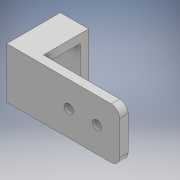
# Autodesk Inventor part: Wheel Holder Rev 2
Saved by Autodesk Inventor 2018 (Build 220112000, 112)
## iProperties
Created: 2018-05-04
Part Number: Wheel Holder Rev 2
Material: Generic
Document SubType Name: Modeling
Designer: alexs
Density: 1 g/cm^3
Appearance: Default
Author: alexs
Autodesk Inventor part; units mm, degrees
ref_plane "YZ Plane" through (0, 0, 0) normal (1, 0, 0) x (0, 1, 0)
ref_plane "XZ Plane" through (0, 0, 0) normal (0, 1, 0) x (-1, 0, 0)
ref_plane "XY Plane" through (0, 0, 0) normal (0, 0, 1) x (1, 0, 0)
sketch "Sketch1" plane through (0, 0, 0) normal (1, 0, 0) x (0, 1, 0)
  line L0 (0, 0) -> (10, 0)
  line L1 (10, 0) -> (10, -12)
  line L2 (10, -12) -> (0, -12)
  line L3 (0, -12) -> (0, 0)
  line L4 (13, 3) -> (-6, 3)
  line L5 (-6, 3) -> (-6, -15)
  line L6 (-6, -15) -> (13, -15)
  line L7 (13, -15) -> (13, 3)
  dimension "d0" = 10
  dimension "d1" = 12
  dimension "d2" = 3
  dimension "d3" = 3
  dimension "d4" = 6
  dimension "d5" = 3
  constraints: 16 end point, 4 parallel, 2 horizontal, 2 perpendicular
  measures "d0" distance of L1.end L2.end
  measures "d1" distance of L0.end L1.end
  measures "d2" distance between parallel lines of L7 L1
  measures "d3" distance between parallel lines of L6 L2
  measures "d4" distance between parallel lines of L3 L5
  measures "d5" distance between parallel lines of L0 L4
extrude "Extrusion1" add sketch "Sketch1" along normal blind 10
sketch "Sketch2" plane through (10, 0, 0) normal (1, 0, 0) x (0, 0, -1)
  line L0 (15, -6) -> (15, 13) construction
  line L1 (-3, -6) -> (15, -6) construction
  line L2 (-3, 13) -> (-3, -6) construction
  line L3 (15, -6) -> (15, 13) projected
  line L4 (-3, -6) -> (15, -6)
  line L5 (15, -6) -> (15, -3)
  line L6 (15, -3) -> (-3, -3)
  line L7 (-3, -3) -> (-3, -6)
  point P0 (0, 0)
  dimension "d8" = 3
  constraints: 8 end point, 2 parallel, 1 horizontal, 1 perpendicular, 1 point on line
  measures "d8" distance between parallel lines of L1 L6
extrude "Extrusion2" add sketch "Sketch2" along normal blind 30
sketch "Sketch3" plane through (10, -3, 3) normal (0, 1, 0) x (1, 0, 0)
  circle A0 centre (12, 9) radius 1.6
  circle A1 centre (22, 9) radius 1.6
  line L0 (0, 18) -> (30, 18) projected
  line L1 (0, 0) -> (30, 0) projected
  line L2 (30, 18) -> (30, 0) projected
  point P0 (-10, 3)
  dimension "d11" = 3.2
  dimension "d12" = 3.2
  dimension "d13" = 9
  dimension "d14" = 9
  dimension "d15" = 8
  dimension "d16" = 10
  constraints: 2 centre point
  measures "d11" diameter of A0
  measures "d12" diameter of A1
  measures "d13" distance from line of L0 A1.centre
  measures "d14" distance from line of L1 A0.centre
  measures "d15" distance from line of L2 A1.centre
  measures "d16" distance of A0.centre A1.centre
extrude "Extrusion3" cut sketch "Sketch3" against normal through all
fillet "Fillet1" radius 3 2 edges at (40, -4.5, 3) (40, -4.5, -15)
equation "\"d3\" = d2"
equation "\"d4\" = 2 * d2"
equation "\"d5\" = d2"
body "Solid1"
